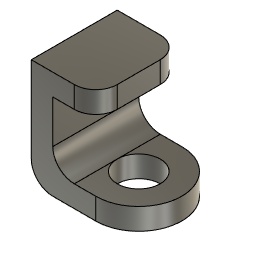
exercise 3 v1 (Autodesk Fusion 360 design; units mm, degrees)
Autodesk Fusion 360 part; units mm, degrees
sketch "Sketch1" plane through (0, 0, 0) normal (0, 1, 0) x (1, 0, 0)
  line L0 (0, 0) -> (-30, 0)
  line L1 (-30, 0) -> (-30, -50)
  line L2 (-30, -50) -> (0, -50)
  line L3 (0, -50) -> (0, -40)
  line L4 (0, -40) -> (-20, -40)
  line L5 (-20, -40) -> (-20, -10)
  line L6 (-20, -10) -> (0, -10)
  line L7 (0, -10) -> (0, 0)
  dimension "d1" = 10
  dimension "d2" = 10
  dimension "d3" = 50
  dimension "d4" = 30
  dimension "d5" = 10
  dimension "d6" = 20
  constraint coincident L0.start L7.end
  constraint horizontal L0
  constraint perpendicular L0 L1
  constraint perpendicular L1 L2
  constraint perpendicular L2 L3
  constraint perpendicular L1 L4
  constraint perpendicular L4 L5
  constraint perpendicular L5 L6
  constraint perpendicular L0 L7
  measures "d1" distance of L2.end L3.end
  measures "d2" distance of L6.end L0.start
  measures "d3" distance of L0.end L1.end
  measures "d4" distance of L1.end L2.end
  measures "d5" distance of L1 L5
  measures "d6" distance of L5.end L6.end
extrude "Extrude1" add sketch "Sketch1" along normal mid plane 40
sketch "Sketch2" plane through (0, 0, 0) normal (0, 0, -1) x (1, 0, 0)
  line L0 (-30, 20) -> (-30, -20)
  line L1 (-30, -20) -> (0, -20)
  line L2 (0, -20) -> (0, 20)
  line L3 (0, 20) -> (-30, 20)
  circle A0 centre (0, 0) radius 20
  circle A1 centre (0, 0) radius 10
  dimension "d9" = 20
  constraint coincident A0.centre A1.centre
  constraint coincident L2.end A0
  constraint concentric A0 A1
  measures "d9" diameter of A1
extrude "Extrude2" add sketch "Sketch2" against normal blind 10 contours L2 A0 A1 picked at (16.5649, -1.4231)
extrude "Extrude3" cut sketch "Sketch2" against normal blind 15 contours L2 A1 picked at (-3.2498, -0.7417)
fillet "Fillet1" radius 10 2 edges at (-20, 0, 10) (-30, 0, 0)
fillet "Fillet2" radius 10 2 edges at (0, -20, 45) (0, 20, 45)
